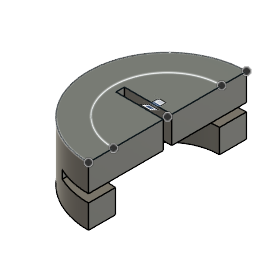
Plunger Guide (Autodesk Fusion 360 design; units mm, degrees)
part number: 2026-05-27-11-56-59-596
Autodesk Fusion 360 part; units mm, degrees
sketch "Sketch1" plane through (0, 0, 0) normal (0, 1, 0) x (1, 0, 0)
  arc A0 (0, 15.375) -> (0, -15.375) centre (0, 0) ccw
  line L0 (0, 15.375) -> (0, 23.375)
  line L1 (0, -15.375) -> (0, -23.375)
  arc A1 (0, 23.375) -> (0, -23.375) centre (0, 0) ccw
  dimension "d1" = 15.375
  dimension "d2" = 8
  constraint coincident A0.centre A1.centre
  constraint vertical A0.end A0.centre
  constraint vertical A0.start A0.centre
  constraint vertical L0
  constraint vertical L1
  constraint equal L0 L1
  measures "d1" radius of A0
  measures "d2" distance of A0.end L1.end
extrude "Extrude1" add sketch "Sketch1" along normal blind 7
sketch "Sketch2" plane through (0, 7, 0) normal (0, 1, 0) x (-1, 0, 0)
  line L0 (0, -15.375) -> (0, -23.375)
  arc A0 (0, -23.375) -> (0, 23.375) centre (0, 0) ccw
  line L1 (0, 23.375) -> (0, 15.375)
  arc A1 (0, -15.375) -> (0, 15.375) centre (0, 0) ccw
  arc A2 (10, -18.937) -> (10, 18.937) centre (-10.625, 0) ccw
  line L2 (17.375, 0) -> (15.375, 0) construction
  line L3 (10, 18.937) -> (10, 21.128)
  line L4 (10, -18.937) -> (10, -21.128)
  arc A3 (10, -21.128) -> (10, 21.128) centre (0, 0) ccw
  dimension "d5" = 2
  dimension "d6" = 28
  dimension "d7" = 10
  constraint midpoint A2 L2.start
  constraint midpoint A1 L2.end
  constraint horizontal L2
  constraint vertical A2.start A2.end
  constraint coincident A0 L3.end
  constraint vertical L3
  constraint coincident A0 L4.end
  constraint vertical L4
  constraint coincident A0.centre A1.centre
  measures "d5" distance of L2.start L2.end
  measures "d6" radius of A2
  measures "d7" distance of L0 A2.start
extrude "Extrude2" add sketch "Sketch2" along normal blind 2.4 contours A0 A2 L3 L4 A3
sketch "Sketch3" plane through (0, 9.4, 0) normal (0, 1, 0) x (-1, 0, 0)
  line L0 (10, -18.937) -> (10, -21.128)
  arc A0 (10, -21.128) -> (10, 21.128) centre (0, 0) ccw
  line L1 (10, 21.128) -> (10, 18.937)
  arc A1 (10, -18.937) -> (10, 18.937) centre (-10.625, 0) ccw
  arc A2 (0, -23.375) -> (0, 23.375) centre (0, 0) ccw
  line L2 (0, -23.375) -> (0, 23.375)
  constraint coincident A0.centre A2.centre
  constraint vertical A2.start A2.end
  constraint equal A0 A2
  constraint coincident A0.centre L2
extrude "Extrude3" add sketch "Sketch3" along normal blind 8
sketch "Sketch4" plane through (0, 17.4, 0) normal (0, 1, 0) x (-1, 0, 0)
  arc A0 (0, -23.375) -> (0, 23.375) centre (0, 0) ccw
  line L0 (0, 23.375) -> (0, -23.375)
  line L1 (0, 0) -> (23.375, 0) construction
  line L2 (0, -1.25) -> (14, -1.25)
  line L3 (14, -1.25) -> (14, 1.25)
  line L4 (14, 1.25) -> (0, 1.25)
  line L5 (0, 1.25) -> (0, -1.25)
  dimension "d17" = 2.5
  dimension "d18" = 14
  constraint coincident A0.centre L1.start
  constraint midpoint A0 L1.end
  constraint horizontal L2
  constraint vertical L3
  constraint horizontal L4
  constraint vertical L5
  constraint coincident L0 L2.start
  constraint midpoint A0.centre L5
  measures "d17" distance of L2.end L3.end
  measures "d18" distance of L2.start L2.end
extrude "Extrude4" cut sketch "Sketch4" against normal through all contours L0 L2 L3 L4 L5
sketch "Sketch5" plane through (0, 17.4, 0) normal (0, 1, 0) x (-1, 0, 0)
  line L0 (14, -1.25) -> (0, -1.25)
  line L1 (0, -1.25) -> (0, -23.375)
  arc A0 (0, -23.375) -> (0, 23.375) centre (0, 0) ccw
  line L2 (0, 23.375) -> (0, 1.25)
  line L3 (0, 1.25) -> (14, 1.25)
  line L4 (14, 1.25) -> (14, -1.25)
  arc A1 (0, -16) -> (0, 16) centre (0, 0) ccw
  arc A2 (0, -23.375) -> (0, 23.375) centre (0, 0) ccw
  dimension "d19" = 16
  constraint coincident L2 A1.end
  constraint coincident L1 A1.start
  constraint coincident A0.centre A1.centre
  constraint coincident A0.end L2.start
  constraint coincident L1.end A0.start
  measures "d19" radius of A1
equation "d1 = ( 30.75 / 2 ) * 1 mm"
